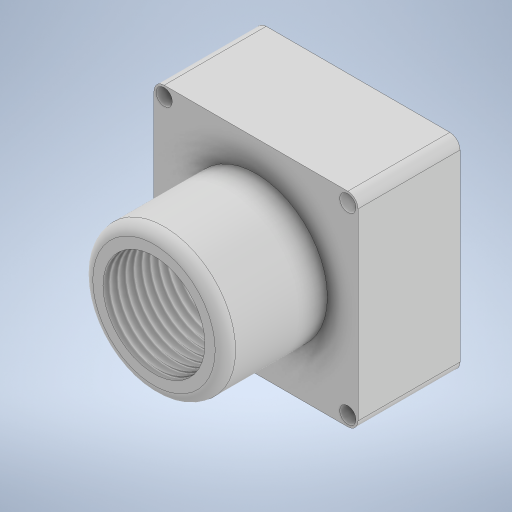
# Autodesk Inventor part: Tarea1
Saved by Autodesk Inventor 2024 (Build 280153000, 153)
## iProperties
Created: 2024-02-19
Part Number: Tarea1
Material: Generic
Document SubType Name: Modeling
Designer: estua
Density: 1 g/cm^3
Appearance: Default
Author: estua
Autodesk Inventor part; units mm, degrees
ref_plane "YZ Plane" through (0, 0, 0) normal (1, 0, 0) x (0, 1, 0)
ref_plane "XZ Plane" through (0, 0, 0) normal (0, 1, 0) x (-1, 0, 0)
ref_plane "XY Plane" through (0, 0, 0) normal (0, 0, 1) x (1, 0, 0)
sketch "Sketch1" plane through (0, 0, 0) normal (0, 0, 1) x (1, 0, 0)
  line L0 (0, 0) -> (100, 0)
  line L1 (100, 0) -> (100, 100)
  line L2 (100, 100) -> (0, 100)
  line L3 (0, 100) -> (0, 0)
  dimension "d0" = 100
  dimension "d1" = 100
  constraints: 8 end point, 2 parallel, 1 horizontal, 1 perpendicular
  measures "d0" distance of L2.end L1.end
  measures "d1" distance of L1.end L0.end
extrude "Extrusion1" add sketch "Sketch1" along normal blind 50
sketch "Sketch2" plane through (0, 0, 50) normal (0, 0, 1) x (1, 0, 0)
  line L0 (100, 100) -> (0, 100) projected
  line L1 (50, 100) -> (50, 0)
  line L2 (0, 100) -> (0, 0) projected
  line L3 (0, 50) -> (100, 50)
  circle A0 centre (50, 50) radius 35
  dimension "d4" = 70
  constraints: 4 end point, 3 midpoint, 1 centre point, 1 horizontal, 1 vertical
  measures "d4" diameter of A0
extrude "Extrusion2" add sketch "Sketch2" along normal blind 50 contours A0 L3 L1 | L1 L3 A0 | L3 A0 L1 | L1 A0 L3
fillet "Fillet1" radius 5 4 edges at (100, 100, 25) (0, 100, 25) (0, 0, 25) (100, 0, 25)
sketch "Sketch3" plane through (50, 50, 100) normal (0, 0, 1) x (1, 0, 0)
  circle A0 centre (0, 0) radius 25
  point P0 (-50, -50)
  dimension "d8" = 50
  constraints: 1 centre point
  measures "d8" diameter of A0
extrude "Extrusion3" cut sketch "Sketch3" against normal blind 100
fillet "Fillet2" radius 5 1 edges at (15, 50, 100)
sketch "Sketch4" plane through (0, 0, 50) normal (0, 0, 1) x (1, 0, 0)
  arc A0 (0, 5) -> (5, 0) centre (5, 5) ccw construction
  circle A1 centre (5, 5) radius 4
  arc A2 (95, 0) -> (100, 5) centre (95, 5) ccw projected
  circle A3 centre (95, 5) radius 4
  arc A4 (100, 95) -> (95, 100) centre (95, 95) ccw projected
  circle A5 centre (95, 95) radius 4
  arc A6 (5, 100) -> (0, 95) centre (5, 95) ccw projected
  circle A7 centre (5, 95) radius 4
  point P0 (0, 0)
  constraints: 4 centre point, 4 coincident
extrude "Extrusion4" cut sketch "Sketch4" against normal blind 100
thread "Thread1" size "M50x4" class "6H" standard "ANSI Metric M Profile" full length
body "Solid1"
